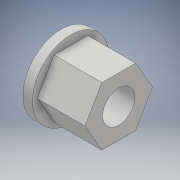
# Autodesk Inventor part: smallHub 9-28
Saved by Autodesk Inventor 2018 (Build 220112000, 112)
## iProperties
Created: 2019-09-28
Part Number: smallHub 9-28
Material: Generic
Document SubType Name: Modeling
Designer: Aditya Kendre
Density: 1 g/cm^3
Appearance: Default
Author: Aditya Kendre
Autodesk Inventor part; units mm, degrees
ref_plane "YZ Plane" through (0, 0, 0) normal (1, 0, 0) x (0, 1, 0)
ref_plane "XZ Plane" through (0, 0, 0) normal (0, 1, 0) x (-1, 0, 0)
ref_plane "XY Plane" through (0, 0, 0) normal (0, 0, 1) x (1, 0, 0)
sketch "Sketch1" plane through (0, 0, 0) normal (1, 0, 0) x (0, 1, 0)
  line L0 (0, 0) -> (0, 6.1) construction
  line L1 (3.5218, 6.1) -> (7.0437, 0)
  line L2 (7.0437, 0) -> (3.5218, -6.1)
  line L3 (3.5218, -6.1) -> (-3.5218, -6.1)
  line L4 (-3.5218, -6.1) -> (-7.0437, 0)
  line L5 (-7.0437, 0) -> (-3.5218, 6.1)
  line L6 (-3.5218, 6.1) -> (3.5218, 6.1)
  dimension "d0" = 6.1
  constraints: 14 end point, 1 coincident, 1 midpoint, 1 vertical, 13 other
  measures "d0" distance of L0.start L0.end
extrude "Extrusion1" add sketch "Sketch1" along normal blind 10
sketch "Sketch2" plane through (0, 0, 0) normal (-1, 0, 0) x (0, 0, 1)
  circle A0 centre (0, 0) radius 3.375
  circle A1 centre (0, 0) radius 8
  dimension "d3" = 6.75
  dimension "d4" = 16
  constraints: 3 coincident, 2 centre point
  measures "d3" diameter of A0
  measures "d4" diameter of A1
extrude "Extrusion2" add sketch "Sketch2" along normal blind 2
sketch "Sketch3" plane through (0, 0, 0) normal (-1, 0, 0) x (0, 0, 1)
  circle A0 centre (0, 0) radius 3.375
  constraints: 1 centre point, 1 coincident
extrude "Extrusion3" cut sketch "Sketch3" against normal blind 10
body "Solid1"
